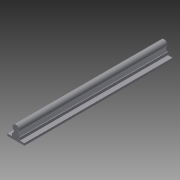
# Autodesk Inventor part: sbr16_350mm
Saved by Autodesk Inventor 2014 (Build 180170000, 170)
## iProperties
Created: 2014-08-13
Part Number: sbr16_350mm
Material: Generic
Document SubType Name: Modeling
Designer: Matthew
Density: 1 g/cm^3
Appearance: Default
Author: Matthew
Autodesk Inventor part; units mm, degrees
ref_plane "YZ Plane" through (0, 0, 0) normal (1, 0, 0) x (0, 1, 0)
ref_plane "XZ Plane" through (0, 0, 0) normal (0, 1, 0) x (-1, 0, 0)
ref_plane "XY Plane" through (0, 0, 0) normal (0, 0, 1) x (1, 0, 0)
sketch "Sketch1" plane through (0, 0, 0) normal (0, 0, 1) x (1, 0, 0)
  line L0 (-20, 0) -> (20, 0)
  line L1 (-20, 0) -> (-20, 5)
  line L2 (20, 0) -> (20, 5)
  line L3 (-20, 5) -> (-9.25, 5)
  line L4 (20, 5) -> (9.25, 5)
  line L5 (-9.25, 5) -> (-9.25, 11.7)
  line L6 (9.25, 5) -> (9.25, 11.7)
  line L7 (-9.25, 5) -> (9.25, 5) construction
  line L8 (-9.25, 5) -> (-4.2961, 5) construction
  line L9 (9.25, 5) -> (3.3755, 5) construction
  arc A0 (4.1601, 14.485) -> (5.7961, 15.0092) centre (4, 17.8) ccw construction
  line L10 (7.926, 11.7) -> (9.25, 11.7)
  line L11 (-7.926, 11.7) -> (-9.25, 11.7)
  arc A1 (3.8717, 17.9993) -> (-3.8717, 17.9993) centre (0, 25) ccw
  line L12 (-3.8717, 17.9993) -> (-7.926, 11.7)
  line L13 (3.8717, 17.9993) -> (7.926, 11.7)
  point P0 (0, 0)
  point P1 (0, 0)
  point P2 (0, 17.8)
  point P3 (0, 5)
  point P4 (-4, 17.8)
  dimension "d0" = 40
  dimension "d1" = 5
  dimension "d2" = 5
  dimension "d3" = 10.75
  dimension "d4" = 10.75
  dimension "d5" = 6.7
  dimension "d6" = 6.7
  dimension "d15" = 25
  dimension "d16" = 18.5
  dimension "d18" = 8
  constraints: 28 end point, 4 coincident, 4 equal length, 4 point on circle, 3 perpendicular, 2 centre point, 2 midpoint, 2 point on line, 1 horizontal, 1 vertical alignment
  measures "d0" distance of L0.start L0.end
  measures "d1" distance of L0.start L1.end
  measures "d2" distance of L0.end L2.end
  measures "d3" distance of L1.end L3.end
  measures "d4" distance of L2.end L4.end
  measures "d5" distance of L3.end L5.end
  measures "d6" distance of L4.end L6.end
  measures "d15" distance from line of L0 point (0, 25)
  measures "d16" distance of L3.end L4.end
  measures "d18" radius of A1
extrude "Extrusion1" add sketch "Sketch1" against normal blind 350
equation "\"d1\" = d2"
equation "\"d3\" = d4"
equation "\"d5\" = d6"
body "Solid1"
